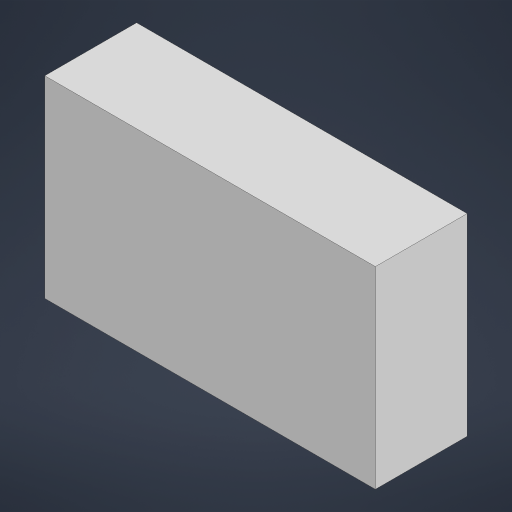
# Autodesk Inventor part: Kypom_K6_7.4V_200mAh_30C60C
Saved by Autodesk Inventor 2023 (Build 270158000, 158)
## iProperties
Created: 2024-06-22
Part Number: Kypom_K6_7.4V_200mAh_30C60C
Material: 一般
Document SubType Name: Modeling
Designer: MasakatsuHonda
Density: 1 g/cm^3
Appearance: 既定
Author: MasakatsuHonda
Autodesk Inventor part; units mm, degrees
ref_plane "YZ Plane" through (0, 0, 0) normal (1, 0, 0) x (0, 1, 0)
ref_plane "XZ Plane" through (0, 0, 0) normal (0, 1, 0) x (-1, 0, 0)
ref_plane "XY Plane" through (0, 0, 0) normal (0, 0, 1) x (1, 0, 0)
sketch "スケッチ1" plane through (0, 0, 0) normal (0, 0, 1) x (1, 0, 0)
  line L0 (-18, 10.5) -> (18, 10.5)
  line L1 (18, 10.5) -> (18, -10.5)
  line L2 (18, -10.5) -> (-18, -10.5)
  line L3 (-18, -10.5) -> (-18, 10.5)
  line L4 (-18, -10.5) -> (18, 10.5) construction
  line L5 (-18, 10.5) -> (18, -10.5) construction
  point P0 (0, 0)
  point P1 (0, 0)
  dimension "d0" = 21
  dimension "d1" = 36
  constraints: 12 end point, 2 parallel, 1 coincident, 1 horizontal, 1 midpoint, 1 perpendicular
  measures "d0" distance of L2.end L0.start
  measures "d1" distance of L0.start L0.end
extrude "押し出し1" add sketch "スケッチ1" along normal blind 10
